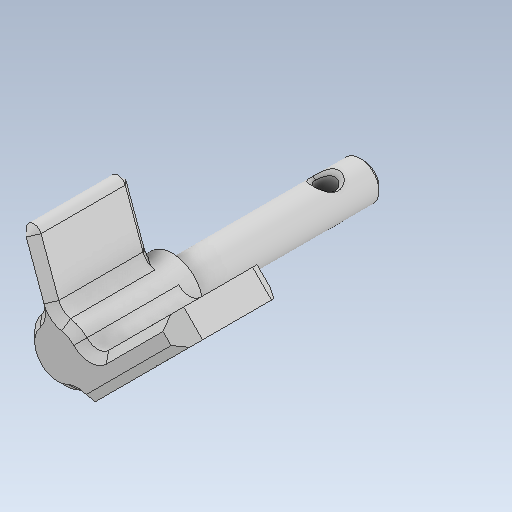
# Autodesk Inventor part: ВнутрНатяжитель
Saved by Autodesk Inventor 2020 (Build 240168000, 168)
## iProperties
Created: 2021-04-26
Part Number: ВнутрНатяжитель
Material: Типовые
Document SubType Name: Modeling
Designer: I_Love_U_Bogdan
Density: 1 g/cm^3
Appearance: По умолчанию
Author: I_Love_U_Bogdan
Autodesk Inventor part; units mm, degrees
ref_plane "YZ Plane" through (0, 0, 0) normal (1, 0, 0) x (0, 1, 0)
ref_plane "XZ Plane" through (0, 0, 0) normal (0, 1, 0) x (-1, 0, 0)
ref_plane "XY Plane" through (0, 0, 0) normal (0, 0, 1) x (1, 0, 0)
sketch "Эскиз1" plane through (0, 0, 0) normal (0, 0, 1) x (1, 0, 0)
  circle A0 centre (0, 0) radius 2.5 projected
  circle A1 centre (0, 0) radius 4
  dimension "d0" = 8
  constraints: 1 centre point, 1 coincident
  measures "d0" diameter of A1
extrude "Выдавливание1" add sketch "Эскиз1" along normal blind 15 contours A0 | A1
sketch "Эскиз2" plane through (0, 0, 15) normal (0, 0, 1) x (1, 0, 0)
  circle A0 centre (15.273549, -186.153338) radius 2.5
  circle A1 centre (19.281341, -181.688183) radius 2.5
  circle A2 centre (6.716372, -177.69288) radius 2.5
  circle A3 centre (6.716372, -107.69288) radius 2.5
  circle A4 centre (11.265758, -120.618493) radius 2.5
  circle A5 centre (6.716372, -37.69288) radius 2.5
  circle A6 centre (15.273549, -46.153338) radius 2.5
  circle A7 centre (23.289132, -37.223028) radius 2.5
  circle A8 centre (26, -154.711547) radius 6
  circle A9 centre (26, -84.711547) radius 6
  circle A10 centre (-32.5, -91.358984) radius 1.5
  circle A11 centre (-32.5, -21.358984) radius 1.5
  line L0 (15.539504, 14.12529) -> (7.458403, 6.044189)
  arc A12 (6.044189, 7.458403) -> (7.458403, 6.044189) centre (0, 0) ccw
  line L1 (6.044189, 7.458403) -> (14.12529, 15.539504)
  arc A13 (14.12529, 15.539504) -> (-20.971241, 1.09865) centre (0, 0) ccw
  arc A14 (-25.052574, -8.068412) -> (-20.971241, 1.09865) centre (-34.952069, 1.831083) ccw
  line L2 (-25.052574, -8.068412) -> (-27.881001, -10.896839)
  line L3 (-27.881001, -5.239985) -> (-27.881001, -10.896839)
  line L4 (-36.464466, -13.82345) -> (-27.881001, -5.239985)
  line L5 (-39, -19.94477) -> (-36.464466, -13.82345)
  line L6 (-39, -107.993214) -> (-39, -19.94477)
  line L7 (-38.705905, -110.227089) -> (-39, -107.993214)
  line L8 (-11.294095, -212.529355) -> (-38.705905, -110.227089)
  line L9 (-10, -222.358984) -> (-11.294095, -212.529355)
  line L10 (-10, -239.530557) -> (-10, -222.358984)
  line L11 (-5.9, -243.630557) -> (-10, -239.530557)
  line L12 (-5.9, -232.316848) -> (-5.9, -243.630557)
  line L13 (-5.9, -232.316848) -> (-1.45329, -236.763558)
  arc A15 (-0.327427, -237.889422) -> (-1.45329, -236.763558) centre (0.635456, -235.800676) ccw
  line L14 (-0.327427, -237.889422) -> (0.141883, -238.358731)
  line L15 (0.141883, -238.358731) -> (21.818108, -232.550604)
  arc A16 (21.818108, -232.550604) -> (28.981437, -229.431762) centre (15, -207.10508) ccw
  arc A17 (32.60983, -226.697303) -> (28.981437, -229.431762) centre (30.579156, -227.777286) ccw
  arc A18 (32.60983, -226.697303) -> (41.343146, -207.10508) centre (15, -207.10508) ccw
  line L16 (41.343146, -207.10508) -> (41.343146, -44.327512)
  line L17 (40.870784, -43.283432) -> (41.343146, -44.327512)
  line L18 (40.870784, -43.283432) -> (30.446504, -37.264971)
  spline S0 degree 3 poles (30.446504, -37.264971) (28.525892, -36.156105) (26.869292, -34.698837) (23.957468, -31.04258) (22.820073, -28.857248) (21.634107, -25.542643) (21.333808, -24.517393) (21.084144, -23.477208) knots -1.71755994 -1.71755994 -1.71755994 -1.71755994 -1.05224042 -1.05224042 -0.31779106 -0.31779106 0 0 0 0
  arc A19 (20.379179, -6.380343) -> (21.084144, -23.477208) centre (25.999994, -14.711543) ccw
  spline S1 degree 3 poles (20.379179, -6.380343) (20.496786, -5.209815) (20.638321, -4.048784) (20.798051, -2.905351) knots 0 0 0 0 1 1 1 1
  arc A20 (20.798051, -2.905351) -> (15.539504, 14.12529) centre (0, 0) ccw
  circle A21 centre (19.281341, -41.688183) radius 2.5
  circle A22 centre (11.265758, -50.618493) radius 2.5
  circle A23 centre (19.281341, -111.688183) radius 2.5
  circle A24 centre (15.273549, -116.153338) radius 2.5
  circle A25 centre (23.289132, -107.223028) radius 2.5
  circle A26 centre (23.289132, -177.223028) radius 2.5
  circle A27 centre (11.265758, -190.618493) radius 2.5
  circle A28 centre (11.595611, -216.817131) radius 12.85
  circle A29 centre (-7.387935, -205.856975) radius 2.3
  circle A30 centre (22.555766, -197.833585) radius 2.3
  circle A31 centre (0, 0) radius 4
  line L19 (3.863703, 1.035276) -> (16.195959, 13.367532)
  line L20 (2.828427, -2.828427) -> (17.405807, 11.748953)
  line L21 (14.470305, 11.641878) -> (15.884519, 10.227664)
  line L22 (0, 0) -> (-4.104242, 11.276311) construction
  line L23 (0.939693, 0.34202) -> (-3.164549, 11.618332)
  line L24 (-5.043934, 10.934291) -> (-0.939693, -0.34202)
  arc A32 (-0.939693, -0.34202) -> (0.939693, 0.34202) centre (0, 0) ccw
  arc A33 (-3.164549, 11.618332) -> (-5.043934, 10.934291) centre (-4.104242, 11.276311) ccw
  point P0 (-2.052121, 5.638156)
  dimension "d3" = 1
  dimension "d4" = 2
  dimension "d5" = 15
  dimension "d6" = 2
  dimension "d7" = 65
  dimension "d8" = 12
  constraints: 14 end point, 8 point on circle, 4 tangent, 3 parallel, 2 centre point, 2 point on line, 1 midpoint, 1 perpendicular
  measures "d3" distance between parallel lines of L0 L19
  measures "d4" distance between parallel lines of L19 L20
  measures "d5" distance from line of L21 L19.start
  measures "d6" diameter of A33
  measures "d7" angle of L19 L22
  measures "d8" distance of L24.start L24.end
extrude "Выдавливание2" add sketch "Эскиз2" against normal blind 13 contours L19 L21 L20 A12 | A12 L20 A31 L19 | L24 A33 L23 A12 | A12 L23 A31 L24 | L23 A32 L24 A31 picked at (-0.349005, 1.286846)
sketch "Эскиз3" plane through (2.828427, -2.828427, 15) normal (0.7071068, -0.7071068, 0) x (-0.7071068, -0.7071068, 0)
  circle A0 centre (-14.442753, 8.8) radius 1.5
  circle A1 centre (-14.442753, 3.8) radius 1.5
  line L0 (-11.542753, 2.125684) -> (-14.442753, 0.451368)
  line L1 (-14.442753, 0.451368) -> (-17.342753, 2.125684)
  line L2 (-17.342753, 2.125684) -> (-17.342753, 5.474316)
  line L3 (-17.342753, 5.474316) -> (-15.912626, 6.3)
  line L4 (-12.97288, 6.3) -> (-11.542753, 5.474316)
  line L5 (-11.542753, 5.474316) -> (-11.542753, 2.125684)
  line L6 (-11.542753, 7.125684) -> (-12.97288, 6.3)
  line L7 (-15.912626, 6.3) -> (-17.342753, 7.125684)
  line L8 (-17.342753, 7.125684) -> (-17.342753, 10.474316)
  line L9 (-17.342753, 10.474316) -> (-14.442753, 12.148632)
  line L10 (-14.442753, 12.148632) -> (-11.542753, 10.474316)
  line L11 (-11.542753, 10.474316) -> (-11.542753, 7.125684)
  line L12 (-18.464102, 0) -> (-18.464102, 13)
  line L13 (0, 0) -> (-18.464102, 0)
  line L14 (0, 13) -> (0, 0)
  line L15 (-18.464102, 13) -> (0, 13)
  line L16 (-18.464102, 0) -> (-18.464102, 13)
  line L17 (-17.464102, 1) -> (-1, 1)
  line L18 (-1, 1) -> (-1, 12)
  line L19 (-1, 12) -> (-17.464102, 12)
  line L20 (-17.464102, 12) -> (-17.464102, 1)
  line L21 (-10.542753, 1.548334) -> (-13.224546, 0)
  line L22 (-15.66096, 0) -> (-18.342753, 1.548334)
  line L23 (-18.342753, 1.548334) -> (-18.342753, 6.051666)
  line L24 (-18.342753, 6.051666) -> (-16.912626, 6.87735)
  line L25 (-10.542753, 6.051666) -> (-10.542753, 1.548334)
  line L26 (-10.542753, 6.548334) -> (-11.97288, 5.72265)
  line L27 (-18.342753, 6.548334) -> (-18.342753, 11.051666)
  line L28 (-18.342753, 11.051666) -> (-14.96814, 13)
  line L29 (-13.917366, 13) -> (-10.542753, 11.051666)
  line L30 (-10.542753, 11.051666) -> (-10.542753, 6.548334)
  line L31 (-13.442753, 7.725982) -> (-13.413331, 7.708995)
  line L32 (-11.97288, 6.87735) -> (-10.542753, 6.051666)
  line L33 (-15.442753, 4.874018) -> (-15.472174, 4.891005)
  line L34 (-16.912626, 5.72265) -> (-18.342753, 6.548334)
  point P0 (0, 15)
  point P1 (-18.464102, 13)
  point P2 (-18.464102, 0)
  point P3 (-13.492495, 1)
  point P4 (-15.393011, 1)
  point P5 (-17.464102, 6.558956)
  point P6 (-17.464102, 6.041044)
  point P7 (-17.912626, 6.3)
  point P8 (-11.492495, 1)
  point P9 (-10.97288, 6.3)
  point P10 (-12.185315, 12)
  dimension "d11" = 5.8
  dimension "d12" = 1
  dimension "d13" = 1
  dimension "d14" = 1
  constraints: 60 end point, 11 point on line, 2 coincident, 2 parallel, 29 other
  measures "d11" distance between parallel lines of L2 L5
  measures "d12" distance between parallel lines of L13 L17
  measures "d13" distance between parallel lines of L5 L25
  measures "d14" distance between parallel lines of L11 L30
extrude "Выдавливание3" add sketch "Эскиз3" along normal blind 1.5 contours L5 L4 L26 L32 L25 L21 L17 L0 | L17 L21 L13 L22 L1 L0 | L0 L1 L17 | L17 L22 L20 L34 L3 L2 L1 | L17 L18 L19 L29 L15 L14 L13 L21 | L4 L6 L32 L26 | L22 L13 L12 L15 L28 L19 L20 L27 L34 L24 L23 L17 | L17 L20 L22 | L32 L6 L11 L10 L19 L29 L30 L26 | L22 L23 L24 L34 L20 | L34 L20 L24 L7 L3 | L19 L10 L9 L28 L15 L29 | L24 L34 L27 L28 L20 | L20 L28 L19 L9 L8 L7 L24 | L20 L19 L28
chamfer "Фаска1" distance 2 angle 45 2 edges at (15.7077, 10.4044, 15) (15.7077, 10.4044, 2)
sketch "Эскиз4" plane through (15.091605, 9.434751, 12.874316) normal (0.7071068, -0.7071068, 0) x (-0.7071068, -0.7071068, 0)
  circle A0 centre (2.9, 1.674316) radius 1.5
  circle A1 centre (2.9, 6.674316) radius 1.5
  point P0 (17.342753, 12.874316)
extrude "Выдавливание4" cut sketch "Эскиз4" against normal through all
fillet "Сопряжение1" radius 2 4 edges at (2.8284, -2.8284, 8.5) (3.8637, 1.0353, 8.5) (-0.3849, 3.9814, 8.5) (-2.2643, 3.2974, 8.5)
chamfer "Фаска2" distance 1 angle 45 17 edges at (9.71, 1.9319, 15) (9.71, 1.9319, 2) (1.847, 3.548, 15) (-0.2437, 4.3768, 15) (-2.001, 8.4216, 15) (-4.4463, 12.216, 15) (-3.8804, 7.7375, 15) (-2.6267, 3.5094, 15) (-3.1608, -2.4514, 15) (2.8502, -3.4281, 15) (4.2426, 2.2426, 15) (9.3565, 6.528, 15) (-3.8804, 7.7375, 2) (-4.4463, 12.216, 2) (-2.001, 8.4216, 2) (-0.2437, 4.3768, 2) (-2.6267, 3.5094, 2)
chamfer "Фаска3" distance 1.5 angle 45 2 edges at (7.4901, 1.8333, 3) (7.2452, 1.5883, 14)
sketch "Эскиз5" plane through (0, 0, 0) normal (0, 0, -1) x (-1, 0, 0)
  circle A0 centre (0, 0) radius 4 projected
  circle A1 centre (0, 0) radius 2.5
  dimension "d42" = 5
  constraints: 1 centre point, 1 coincident
  measures "d42" diameter of A1
extrude "Выдавливание5" add sketch "Эскиз5" along normal blind 25 contours A1
sketch "Эскиз6" plane through (0, 0, 0) normal (1, 0, 0) x (0, 1, 0)
  line L0 (2.828427, 14) -> (3.939231, 14)
  line L1 (2.828427, 2) -> (2.828427, 14)
  line L2 (2.828427, 2) -> (-3.607543, 2)
  line L3 (-3.607543, 14) -> (-3.607543, 2)
  line L4 (2.57115, 14) -> (-3.607543, 14)
  line L5 (2.57115, 3) -> (2.57115, 14)
  line L6 (3.665013, 2) -> (3.837565, 2)
  line L7 (3.939231, 14) -> (3.939231, 3)
  circle A0 centre (0, -10) radius 1.25
  point P0 (0, 0)
  point P1 (-4, -25)
  point P2 (4, -25)
  dimension "d31" = 2.5
  constraints: 1 centre point, 2 other
  measures "d31" diameter of A0
extrude "Выдавливание6" [suppressed]
sketch "Эскиз7" plane through (0, 0, 0) normal (0, 1, 0) x (-1, 0, 0)
  circle A0 centre (0, -20) radius 1.25
  line L0 (-4, -25) -> (4, -25) projected
  point P0 (0, 0)
  dimension "d38" = 2.5
  dimension "d39" = 5
  constraints: 1 centre point
  measures "d38" diameter of A0
  measures "d39" distance from line of L0 A0.centre
extrude "Выдавливание7" cut sketch "Эскиз7" against normal mid plane 25
chamfer "Фаска4" distance 0.5 angle 45 2 edges at (1.25, -2.1651, -20.0039) (1.25, 2.1651, -20.0039)
chamfer "Фаска5" distance 0.5 angle 45 1 edges at (2.5, 0, -25)
